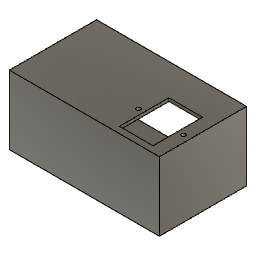
Power_Supply_Cover v2 (Autodesk Fusion 360 design; units mm, degrees)
Autodesk Fusion 360 part; units mm, degrees
sketch "Top" plane through (0, 0, 0) normal (0, 0, 1) x (1, 0, 0)
  line L0 (-60.071, 34.925) -> (60.071, 34.925)
  line L1 (60.071, 34.925) -> (60.071, -34.925)
  line L2 (60.071, -34.925) -> (-60.071, -34.925)
  line L3 (-60.071, -34.925) -> (-60.071, 34.925)
  point P0 (0, 34.925)
  point P1 (60.071, 0)
  dimension "d1" = 69.85
  dimension "d2" = 120.142
  constraint horizontal L0
  constraint vertical L1
  constraint horizontal L2
  constraint vertical L3
  constraint midpoint L0 P0
  constraint vertical origin P0
  constraint midpoint L1 P1
  constraint horizontal origin P1
  measures "d1" distance of L0.start L2.end
  measures "d2" distance of L0.start L0.end
extrude "Extrude2" add sketch "Top" along normal blind 55.118
form "Form1" [no effect]
sketch "Sketch2" plane through (0, 0, 0) normal (0, 0, 1) x (1, 0, 0)
  line L0 (22.987, 9.779) -> (49.911, 9.779)
  line L1 (49.911, 9.779) -> (49.911, -29.845)
  line L2 (49.911, -29.845) -> (22.987, -29.845)
  line L3 (22.987, -29.845) -> (22.987, 9.779)
  circle A0 centre (18.4531, -10.033) radius 1.651
  circle A1 centre (54.4449, -10.033) radius 1.651
  line L4 (60.071, -34.925) -> (-60.071, -34.925)
  line L5 (60.071, 34.925) -> (60.071, -34.925)
  point P0 (22.987, -10.033)
  dimension "d7" = 26.924
  dimension "d8" = 39.624
  dimension "d9" = 5.08
  dimension "d10" = 35.9918
  dimension "d11" = 4.5339
  dimension "d12" = 3.302
  dimension "d13" = 10.16
  constraint horizontal L0
  constraint vertical L1
  constraint horizontal L2
  constraint vertical L3
  constraint horizontal A0.centre A1.centre
  constraint midpoint L3 P0
  constraint horizontal A0.centre P0
  constraint equal A0 A1
  measures "d7" distance of L0.start L0.end
  measures "d8" distance of L0.start L2.end
  measures "d9" distance of L2 L4
  measures "d10" distance of A0.centre A1.centre
  measures "d11" distance of L3 A0.centre
  measures "d12" diameter of A0
  measures "d13" distance of L1 L5
extrude "Extrude3" cut sketch "Sketch2" along normal blind 55.88 and the other way blind -5.08
sketch "Sketch3" plane through (0, 34.925, 0) normal (0, 1, 0) x (-1, 0, 0)
  line L0 (-60.071, 0) -> (60.071, 0)
  line L1 (60.071, 0) -> (60.071, 55.118)
  line L2 (60.071, 55.118) -> (-60.071, 55.118)
  line L3 (-60.071, 55.118) -> (-60.071, 0)
  line L4 (-58.039, 52.578) -> (58.039, 52.578)
  line L5 (58.039, 52.578) -> (58.039, 2.54)
  line L6 (58.039, 2.54) -> (-58.039, 2.54)
  line L7 (-58.039, 2.54) -> (-58.039, 52.578)
  line L8 (-60.071, 0) -> (60.071, 0)
  point P0 (0, 52.578)
  point P1 (0, 55.118)
  point P2 (-58.039, 27.559)
  point P3 (-60.071, 27.559)
  point P4 (-60.071, 0)
  point P5 (60.071, 0)
  dimension "d16" = 116.078
  dimension "d17" = 113.03
  dimension "d18" = 113.03
  dimension "d19" = 50.038
  constraint horizontal L4
  constraint vertical L5
  constraint horizontal L6
  constraint vertical L7
  constraint midpoint L4 P0
  constraint midpoint L2 P1
  constraint midpoint L7 P2
  constraint midpoint L3 P3
  constraint horizontal P2 P3
  constraint vertical P0 P1
  measures "d16" distance of L4.start L4.end
  measures "d19" distance of L4.start L6.end
extrude "Extrude4" cut sketch "Sketch3" against normal blind 65.024 contours L4 L5 L6 L7
